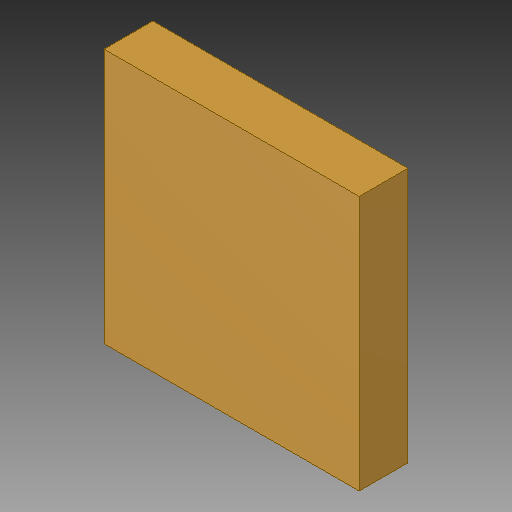
# Autodesk Inventor part: E2-5
Saved by Autodesk Inventor 2017 (Build 210142000, 142)
## iProperties
Created: 2019-06-13
Part Number: E2-5
Material: Generic
Document SubType Name: Modeling
Designer: Marc
Density: 1 g/cm^3
Appearance: E2-5, E2-5
Author: Marc
Autodesk Inventor part; units mm, degrees
ref_plane "YZ Plane" through (0, 0, 0) normal (1, 0, 0) x (0, 1, 0)
ref_plane "XZ Plane" through (0, 0, 0) normal (0, 1, 0) x (-1, 0, 0)
ref_plane "XY Plane" through (0, 0, 0) normal (0, 0, 1) x (1, 0, 0)
sketch "E2-5, E2-5_7" plane through (0, 0, 0) normal (0, 0, 1) x (1, 0, 0)
  line L0 (-2.6162, 2.6162) -> (2.6162, 2.6162)
  line L1 (2.6162, 2.6162) -> (2.6162, -2.6162)
  line L2 (2.6162, -2.6162) -> (-2.6162, -2.6162)
  line L3 (-2.6162, -2.6162) -> (-2.6162, 2.6162)
  constraints: 8 end point
extrude "Extrusion1" add sketch "E2-5, E2-5_7" along normal blind 1
body "Solid1"
